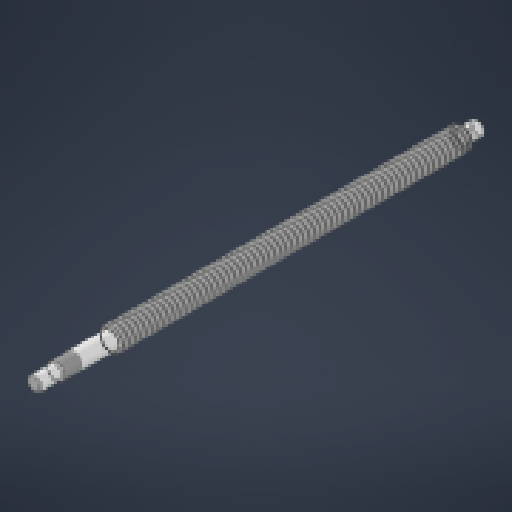
# Autodesk Inventor part: SFU1605_250mm
Saved by Autodesk Inventor 2023 (Build 270158000, 158)
## iProperties
Created: 2025-09-04
Part Number: SFU1605_250mm
Material: 일반
Document SubType Name: Modeling
Designer: k
Density: 1 g/cm^3
Appearance: 기본값
Author: k
Autodesk Inventor part; units mm, degrees
ref_plane "YZ Plane" through (0, 0, 0) normal (1, 0, 0) x (0, 1, 0)
ref_plane "XZ Plane" through (0, 0, 0) normal (0, 1, 0) x (-1, 0, 0)
ref_plane "XY Plane" through (0, 0, 0) normal (0, 0, 1) x (1, 0, 0)
sketch "스케치1" plane through (0, 0, 0) normal (1, 0, 0) x (0, 1, 0)
  line L0 (78.9967, 284.4353) -> (78.9967, -30.5647)
  line L1 (78.9967, 284.4353) -> (83.9967, 284.4353)
  line L2 (83.9967, 284.4353) -> (83.9967, 269.4353)
  line L3 (83.9967, 269.4353) -> (84.9967, 269.4353)
  line L4 (84.9967, 269.4353) -> (84.9967, 230.4353)
  line L5 (84.9967, 230.4353) -> (86.9967, 230.4353)
  line L6 (86.9967, 230.4353) -> (86.9967, -19.5647)
  line L7 (86.9967, -19.5647) -> (83.9967, -19.5647)
  line L8 (83.9967, -19.5647) -> (83.9967, -30.5647)
  line L9 (83.9967, -30.5647) -> (78.9967, -30.5647)
  point P0 (0, 0)
  dimension "d3" = 5
  dimension "d4" = 15
  dimension "d5" = 1
  dimension "d6" = 39
  dimension "d7" = 2
  dimension "d8" = 250
  dimension "d9" = 5
  dimension "d10" = 11
  constraints: 20 end point, 7 perpendicular, 2 vertical, 1 horizontal
  measures "d3" distance of L0.start L1.end
  measures "d4" distance of L1.end L2.end
  measures "d5" distance of L2.end L3.end
  measures "d6" distance of L3.end L4.end
  measures "d7" distance of L4.end L5.end
  measures "d8" distance of L5.end L6.end
  measures "d9" distance of L8.end L0.end
  measures "d10" distance of L7.end L8.end
revolve "회전1" add sketch "스케치1" angle 360 about axis through (0, 78.9967, 284.4353) along (0, 0, -1)
chamfer "모따기1" distance 1 angle 45 2 edges at (0, 73.9967, 284.4353) (0, 73.9967, -30.5647)
thread "스레드1" size "M12x1" class "6g" standard "ANSI Metric M Profile" length 14
thread "스레드2" size "TR16x4" class "7e" standard "ISO Metric Trapezoidal Threads" full length
chamfer "모따기2" distance 1 angle 45 1 edges at (0, 72.9967, 269.4353)
chamfer "모따기3" distance 1 angle 45 2 edges at (0, 70.9967, 230.4353) (0, 70.9967, -19.5647)
